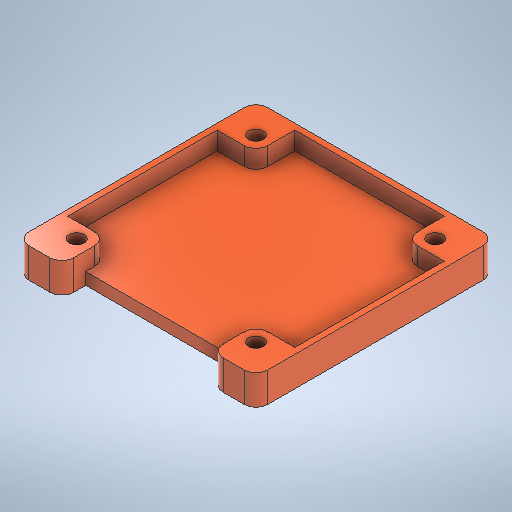
# Autodesk Inventor part: CameraMount2
Saved by Autodesk Inventor 2025 (Build 290162010, 162A)
## iProperties
Created: 2024-07-04
Part Number: CameraMount2
Material: Generic
Document SubType Name: Modeling
Designer: rolan
Density: 1 g/cm^3
Appearance: Default
Author: rolan
Autodesk Inventor part; units mm, degrees
ref_plane "YZ Plane" through (0, 0, 0) normal (1, 0, 0) x (0, 1, 0)
ref_plane "XZ Plane" through (0, 0, 0) normal (0, 1, 0) x (-1, 0, 0)
ref_plane "XY Plane" through (0, 0, 0) normal (0, 0, 1) x (1, 0, 0)
sketch "Sketch1" plane through (0, 0, 0) normal (0, 1, 0) x (-1, 0, 0)
  line L0 (19, 19) -> (-19, 19) construction
  line L1 (-19, 19) -> (-19, -19) construction
  line L2 (-19, -19) -> (19, -19) construction
  line L3 (19, -19) -> (19, 19) construction
  line L4 (19, 19) -> (-19, -19) construction
  line L5 (-19, 19) -> (19, -19) construction
  circle A0 centre (15, -15) radius 1.25
  circle A1 centre (-15, -15) radius 1.25
  circle A2 centre (15, 15) radius 1.25
  circle A3 centre (-15, 15) radius 1.25
  line L6 (20, 20) -> (-20, 20)
  line L7 (-20, 20) -> (-20, -20)
  line L8 (-20, -20) -> (20, -20)
  line L9 (20, -20) -> (20, 20)
  line L10 (20, 20) -> (-20, -20) construction
  line L11 (-20, 20) -> (20, -20) construction
  point P0 (0, 0)
  dimension "d0" = 38
  dimension "d1" = 38
  dimension "d2" = 2.5
  dimension "d3" = 2.5
  dimension "d4" = 2.5
  dimension "d5" = 2.5
  dimension "d6" = 4
  dimension "d7" = 4
  dimension "d8" = 4
  dimension "d9" = 4
  dimension "d10" = 40
  dimension "d11" = 40
  constraints: 24 end point, 4 centre point, 4 midpoint, 4 parallel, 2 horizontal, 2 horizontal alignment, 2 perpendicular, 2 vertical alignment
  measures "d0" distance of L1.end L2.end
  measures "d1" distance of L0.end L1.end
  measures "d2" diameter of A1
  measures "d3" diameter of A0
  measures "d4" diameter of A2
  measures "d5" diameter of A3
  measures "d6" distance from line of L2 A0.centre
  measures "d7" distance from line of L3 A0.centre
  measures "d8" distance from line of L0 A3.centre
  measures "d9" distance from line of L1 A3.centre
  measures "d10" distance of L8.end L7.end
  measures "d11" distance of L7.end L6.end
extrude "Extrusion1" add sketch "Sketch1" along normal blind 5
sketch "Sketch2" plane through (0, 5, 0) normal (0, 1, 0) x (1, 0, 0)
  line L0 (-12.5, 19) -> (-12.5, 12.5)
  line L1 (-12.5, 12.5) -> (-19, 12.5)
  line L2 (-19, 12.5) -> (-19, -12.5)
  line L3 (-20, 20) -> (-20, -20) projected
  line L4 (-19, -12.5) -> (-12.5, -12.5)
  line L5 (-12.5, -12.5) -> (-12.5, -20)
  line L6 (-12.5, -20) -> (12.5, -20)
  line L7 (12.5, -20) -> (12.5, -12.5)
  line L8 (12.5, -12.5) -> (19, -12.5)
  line L9 (19, -12.5) -> (19, 12.5)
  line L10 (19, 12.5) -> (12.5, 12.5)
  line L11 (12.5, 12.5) -> (12.5, 19)
  line L12 (12.5, 19) -> (-12.5, 19)
  point P0 (0, 0)
  dimension "d14" = 25
  dimension "d15" = 6.5
  dimension "d16" = 25
  dimension "d17" = 7.5
  dimension "d18" = 6.5
  dimension "d19" = 6.5
  dimension "d20" = 25
  dimension "d21" = 6.5
  dimension "d22" = 12.5
  dimension "d24" = 12.5
  constraints: 24 end point, 8 perpendicular, 4 point on line, 1 parallel, 1 vertical
  measures "d14" distance of L0.start L11.end
  measures "d15" distance of L10.end L11.end
  measures "d16" distance of L8.end L9.end
  measures "d17" distance between parallel lines of L6 L8
  measures "d18" distance between parallel lines of L9 L11
  measures "d19" distance between parallel lines of L9 L7
  measures "d20" distance of L5.end L6.end
  measures "d21" distance between parallel lines of L2 L5
  measures "d22" horizontal distance of point (0, 0) L0.start
  measures "d24" horizontal distance of point (0, 0) L0.end
extrude "Extrusion2" cut sketch "Sketch2" against normal blind 3
sketch "Sketch3" plane through (0, 2, 0) normal (0, 1, 0) x (1, 0, 0)
  line L0 (12.5, -12.5) -> (12.5, -20) projected
  line L1 (-12.5, -20) -> (12.5, -20)
  line L2 (12.5, -20) -> (12.5, -16)
  line L3 (12.5, -16) -> (-12.5, -16)
  line L4 (-12.5, -16) -> (-12.5, -20)
  point P0 (0, 0)
  dimension "d27" = 4
  constraints: 8 end point, 2 parallel, 1 horizontal, 1 perpendicular, 1 point on line
  measures "d27" distance of L2.end L1.end
extrude "Extrusion3" cut sketch "Sketch3" against normal through all
fillet "Fillet1" radius 2 10 edges at (-20, 2.5, -20) (20, 2.5, -20) (-20, 2.5, 20) (20, 2.5, 20) (-12.5, 3.5, -12.5) (12.5, 3.5, -12.5) (12.5, 3.5, 12.5) (-12.5, 3.5, 12.5) (-12.5, 2.5, 20) (12.5, 2.5, 20)
body "Solid1"
